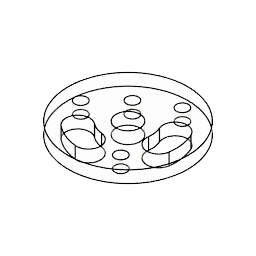
UpperVertibraeV1_v11 (Autodesk Fusion 360 design; units mm, degrees)
Autodesk Fusion 360 part; units mm, degrees
sketch "Sketch1" plane through (0, 0, 0) normal (0, 0, 1) x (1, 0, 0)
  circle A0 centre (0, 0) radius 8
  circle A1 centre (5.4981, 2.4023) radius 2
  line L0 (4.3113, -5.5147) -> (0, 0) construction
  line L1 (0, 0) -> (5.4981, 2.4023) construction
  circle A2 centre (-4.8295, 3.5603) radius 2 construction
  circle A3 centre (-6.9316, -0.9764) radius 1
  circle A4 centre (2.6202, 6.4911) radius 1
  circle A5 centre (0, 0) radius 10
  circle A6 centre (0, 0) radius 4
  circle A7 centre (4.3113, -5.5147) radius 3
  circle A8 centre (2.6202, 6.4911) radius 3
  circle A9 centre (5.9478, -0.7901) radius 2
  circle A10 centre (-2.2896, 5.546) radius 2 construction
  circle A11 centre (4.3113, -5.5147) radius 1
  line L2 (0, 0) -> (-7, 0) construction
  circle A12 centre (-3.6581, -4.7559) radius 2
  line L3 (0, 0) -> (2.6202, 6.4911) construction
  circle A13 centre (0, 0) radius 2
  circle A14 centre (-6.9316, -0.9764) radius 3
  circle A15 centre (-0.6686, -5.9626) radius 2
  line L4 (-4.8295, 3.5603) -> (-2.2896, 5.546) construction
  line L5 (-3.5596, 4.5531) -> (-2.6357, 3.3714) construction
  circle A16 centre (-2.6357, 3.3714) radius 1
  line L6 (-2.6357, 3.3714) -> (0, 0) construction
  dimension "d22" = 360
  dimension "d24" = 360
  dimension "d25" = 20
  dimension "d26" = 4
  dimension "d27" = 7
  dimension "d28" = 8
  dimension "d29" = 7
  dimension "d30" = 2
  dimension "d31" = 16
  dimension "d32" = 6
  dimension "d33" = 6
  dimension "d34" = 120
  dimension "d45" = 1.5
  dimension "d46" = 2
  constraint coincident A0.centre L0.end
  constraint horizontal L2
  constraint concentric A0 A13
  constraint concentric A4 A8
  constraint tangent A6 A8
  constraint coincident A4.centre A8.centre
  constraint coincident A1.centre L1.end
  constraint tangent A1 A6
  constraint tangent A1 A8
  constraint tangent A6 A9
  constraint coincident L0.start A7.centre
  constraint tangent A7 A9
  constraint coincident A2.centre L4.start
  constraint coincident A10.centre L4.end
  constraint midpoint L4 L5.start
  constraint perpendicular L4 L5
  constraint coincident L5.end A16.centre
  measures "d25" diameter of A5
  measures "d26" diameter of A13
  measures "d27" distance of A0.centre L2.end
  measures "d28" diameter of A6
  measures "d29" distance of A4.centre A0.centre
  measures "d30" diameter of A4
  measures "d31" diameter of A0
  measures "d32" distance of A1.centre A0.centre
  measures "d33" distance of A0.centre A9.centre
  measures "d34" angle of L0 L3
  measures "d45" distance of L5.start L5.end
  measures "d46" diameter of A16
extrude "Extrude1" add sketch "Sketch1" along normal blind 2 contours A0 A5 A7 A8 | A0 A1 A8 | A0 A7 A9 | A0 A8 | A0 A8 | A1 A6 A8 | A0 A7 | A0 A7 | A6 A7 A9 | A6 A16 | A0 A6 A8 A14 A16 | A6 A7 A15 | A0 A5 A8 A14 | A0 A5 A7 A14 | A0 A7 A15 | A0 A14 | A0 A14 | A6 A12 A14 | A0 A12 A14 picked at (-2.727, 1.6035)
